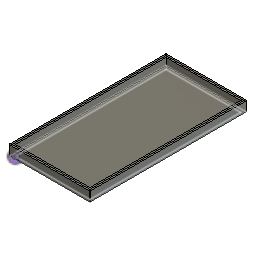
auber cover (Autodesk Fusion 360 design; units mm, degrees)
Autodesk Fusion 360 part; units mm, degrees
sketch "Sketch1" plane through (0, 0, 0) normal (0, 1, 0) x (1, 0, 0)
  line L0 (0, 0) -> (23.5, 0)
  line L1 (23.5, 0) -> (23.5, 47.5)
  line L2 (23.5, 47.5) -> (0, 47.5)
  line L3 (0, 47.5) -> (0, 0)
  line L4 (-1, -1) -> (24.5, -1)
  line L5 (24.5, -1) -> (24.5, 48.5)
  line L6 (24.5, 48.5) -> (-1, 48.5)
  line L7 (-1, 48.5) -> (-1, -1)
  dimension "d1" = 23.5
  dimension "d2" = 47.5
  dimension "d3" = 1
  constraint horizontal L0
  constraint vertical L1
  constraint horizontal L2
  constraint vertical L3
  constraint coincident L0.start L3.end
  measures "d1" distance of L0.start L0.end
  measures "d2" distance of L0.start L2.end
extrude "Extrude1" add sketch "Sketch1" along normal blind 1 contours L0 L1 L2 L3
extrude "Extrude2" add sketch "Sketch1" along normal blind 3.5
fillet "Fillet1" radius 0.25 7 edges at (11.75, 0, 1) (24.5, 0, -23.75) (11.75, 3.5, 1) (0, 3.5, -23.75) (11.75, 3.5, -47.5) (23.5, 3.5, -23.75) (11.75, 3.5, 0) 4 faces at (24.5, 1.1667, -15.5) (16, 1.1667, -48.5) (7.5, 0, -32) (-1, 1.1667, -32)
